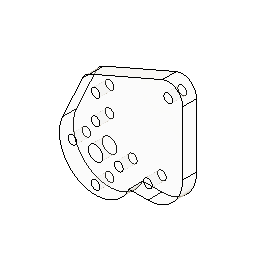
AssemblyHolderThrowerMotor v5 (Autodesk Fusion 360 archive; units mm, degrees)
design "ThrowerMotorJunction"
Autodesk Fusion 360 part; units mm, degrees
sketch "Sketch1" plane through (0, 0, 0) normal (0, 1, 0) x (1, 0, 0)
  circle A0 centre (0, 0) radius 8 construction
  circle A1 centre (0, 0) radius 9.5 construction
  circle A2 centre (0, 0) radius 14 construction
  circle A3 centre (0, 0) radius 18 construction
  line L0 (0, 0) -> (0, -18) construction
  line L1 (0, 0) -> (0, 52) construction
  line L2 (0, 0) -> (18, 0) construction
  line L3 (0, 0) -> (-18, 0) construction
  circle A4 centre (0, 0) radius 48 construction
  circle A5 centre (0, 0) radius 58 construction
  line L4 (0, 47) -> (-33.9853, 47) construction
  circle A6 centre (0, -9.5) radius 1.5
  circle A7 centre (-8, 0) radius 1.5
  circle A8 centre (8, 0) radius 1.5
  circle A9 centre (0, 9.5) radius 1.5
  circle A10 centre (18, 0) radius 1.5
  circle A11 centre (0, -18) radius 1.5
  line L5 (-50.3158, -28.85) -> (25, -28.85) construction
  circle A12 centre (25, -28.85) radius 1.5
  line L6 (-11.3632, -5.2083) -> (-4.1251, -21)
  line L7 (11.4564, 5) -> (18, 5)
  line L8 (30, -7) -> (30, -28.85)
  arc A13 (12.5, 0) -> (11.4564, 5) centre (0, 0) ccw construction
  arc A14 (11.4564, 5) -> (-11.3632, -5.2083) centre (0, 0) ccw
  arc A15 (0, -12.5) -> (12.5, 0) centre (0, 0) ccw construction
  arc A16 (-11.3632, -5.2083) -> (0, -12.5) centre (0, 0) ccw construction
  circle A17 centre (0, 0) radius 2.5
  arc A18 (30, -28.85) -> (23.0094, -33.4367) centre (25, -28.85) ccw construction
  arc A19 (23.0094, -33.4367) -> (30, -28.85) centre (25, -28.85) ccw
  line L9 (-1.9906, -22.5867) -> (23.0094, -33.4367)
  arc A20 (-1.9906, -22.5867) -> (-4.5453, -20.0833) centre (0, -18) ccw construction
  arc A21 (-4.5453, -20.0833) -> (-1.9906, -22.5867) centre (0, -18) ccw
  arc A22 (18, 5) -> (30, -7) centre (18, -7) ccw construction
  arc A23 (30, -7) -> (18, 5) centre (18, -7) ccw
  point P0 (0, 14)
  point P1 (0, 47)
  point P2 (-47.869, 32.75)
  point P3 (-42.1187, 39.875)
  point P4 (-50.8212, 27.95)
  point P5 (-55.4373, -17.05)
  point P6 (-53.7269, -21.85)
  point P7 (-50.3158, -28.85)
  point P8 (0, 9.5)
  point P9 (8, 0)
  point P10 (0, 12.5)
  dimension "d19" = 16
  dimension "d20" = 19
  dimension "d21" = 28
  dimension "d22" = 36
  dimension "d23" = 38
  dimension "d24" = 96
  dimension "d25" = 116
  dimension "d26" = 5
  dimension "d27" = 19.25
  dimension "d28" = 4.8
  dimension "d29" = 7.125
  dimension "d30" = 45
  dimension "d31" = 4.8
  dimension "d32" = 7
  dimension "d33" = 3
  dimension "d34" = 3
  dimension "d35" = 3
  dimension "d36" = 3
  dimension "d37" = 3
  dimension "d38" = 3
  dimension "d39" = 25
  dimension "d40" = 3
  dimension "d41" = 3
  dimension "d44" = 5
  dimension "d45" = 5
  dimension "d48" = 5
  dimension "d49" = 3
  dimension "d50" = 5
  dimension "d51" = 12
  constraint coincident A0.centre A1.centre
  constraint concentric A0 A2
  constraint concentric A1 A3
  constraint coincident A3 L0.end
  constraint vertical L0
  constraint parallel L0 L1
  constraint coincident A3 L2.end
  constraint horizontal L2
  constraint coincident A3 L3.end
  constraint parallel L2 L3
  constraint coincident A2 P0
  constraint coincident L1 P0
  constraint concentric A0 A4
  constraint concentric A3 A5
  constraint coincident L1 P1
  constraint coincident P1 L4.start
  constraint coincident A5 L4.end
  constraint perpendicular L1 L4
  constraint coincident A5 P2
  constraint coincident A5 P3
  constraint coincident A5 P4
  constraint coincident A5 P5
  constraint coincident A5 P6
  constraint coincident A5 P7
  constraint coincident A1 A6.centre
  constraint coincident L0 A6.centre
  constraint coincident A1 P8
  constraint coincident L1 P8
  constraint coincident A0 A7.centre
  constraint coincident L3 A7.centre
  constraint coincident A0 P9
  constraint coincident L2 P9
  constraint coincident P9 A8.centre
  constraint coincident P8 A9.centre
  constraint coincident L2.end A10.centre
  constraint coincident L0.end A11.centre
  constraint coincident P7 L5.start
  constraint horizontal L5
  constraint coincident L5.end A12.centre
  constraint concentric A3 A14
  constraint coincident L1 P10
  constraint coincident P10 A14
  constraint tangent L6 A14
  constraint horizontal L7
  constraint perpendicular L7 L8
  constraint coincident L2 A13.start
  constraint concentric A13 A14
  constraint coincident L0 A15.start
  constraint concentric A14 A15
  constraint concentric A14 A16
  constraint concentric A5 A17
  constraint concentric A12 A18
  constraint tangent L8 A18
  constraint concentric A18 A19
  constraint concentric A11 A20
  constraint tangent L6 A20
  constraint tangent A18 L9
  constraint tangent L9 A20
  constraint coincident L6 A20.end
  constraint concentric A20 A21
  constraint tangent L8 A22
  constraint tangent L7 A22
  constraint concentric A22 A23
  measures "d19" diameter of A0
  measures "d20" diameter of A1
  measures "d21" diameter of A2
  measures "d22" diameter of A3
  measures "d23" distance of L1.end P0
  measures "d24" diameter of A4
  measures "d25" diameter of A5
  measures "d26" distance of L1.end P1
  measures "d27" vertical distance of L1.end P2
  measures "d28" vertical distance of P2 P4
  measures "d29" vertical distance of P2 P3
  measures "d30" vertical distance of P4 P5
  measures "d31" vertical distance of P5 P6
  measures "d32" vertical distance of P6 P7
  measures "d33" diameter of A6
  measures "d34" diameter of A7
  measures "d35" diameter of A8
  measures "d36" diameter of A9
  measures "d37" diameter of A10
  measures "d38" diameter of A11
  measures "d39" horizontal distance of L0.end L5.end
  measures "d40" diameter of A12
  measures "d41" distance of P8 P10
  measures "d44" distance of L2.end L7
  measures "d45" distance of L5.end L8
  measures "d48" diameter of A17
  measures "d49" vertical distance of L6.end L0.end
  measures "d50" radius of A20
  measures "d51" distance of L8 A22.centre
extrude "Extrude1" add sketch "Sketch1" along normal blind 4.8

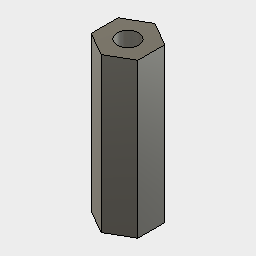
design "Spacer M3x18"
Autodesk Fusion 360 part; units mm, degrees
sketch "Sketch1" plane through (0, 0, 0) normal (0, 1, 0) x (1, 0, 0)
  line L0 (2.725, 1.5733) -> (0, 3.1466)
  line L1 (0, 3.1466) -> (-2.725, 1.5733)
  line L2 (-2.725, 1.5733) -> (-2.725, -1.5733)
  line L3 (-2.725, -1.5733) -> (0, -3.1466)
  line L4 (0, -3.1466) -> (2.725, -1.5733)
  line L5 (2.725, -1.5733) -> (2.725, 1.5733)
  circle A0 centre (0, 0) radius 1.25
  dimension "d1" = 2.5
  measures "d1" diameter of A0
extrude "Extrude1" add sketch "Sketch1" along normal blind 18

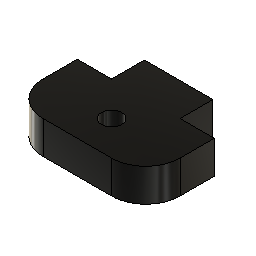
design "ThrowerLock"
Autodesk Fusion 360 part; units mm, degrees
sketch "Sketch1" plane through (0, 0, 0) normal (0, 0, 1) x (1, 0, 0)
  line L0 (-5, 9.8) -> (5, 9.8)
  line L1 (5, 9.8) -> (5, 5)
  line L2 (5, 5) -> (10, 5)
  line L3 (10, 5) -> (10, 0)
  line L4 (5, -5) -> (-5, -5)
  line L5 (-10, 0) -> (-10, 5)
  line L6 (-10, 5) -> (-5, 5)
  line L7 (-5, 5) -> (-5, 9.8)
  line L8 (0, 0) -> (0, 9.8) construction
  line L9 (0, 0) -> (10, 0) construction
  line L10 (0, 0) -> (0, -5) construction
  line L11 (-5, 5) -> (-5, 0) construction
  line L12 (0, 0) -> (-5, 0) construction
  circle A0 centre (0, 0) radius 1.5
  line L13 (-10, -5) -> (-10, 0) construction
  line L14 (-5, -5) -> (-10, -5) construction
  arc A1 (-5, -5) -> (-10, 0) centre (-5, 0) ccw construction
  arc A2 (-10, 0) -> (-5, -5) centre (-5, 0) ccw
  line L15 (10, -5) -> (5, -5) construction
  line L16 (10, 0) -> (10, -5) construction
  arc A3 (10, 0) -> (5, -5) centre (5, 0) ccw construction
  arc A4 (5, -5) -> (10, 0) centre (5, 0) ccw
  point P0 (0, 9.8)
  point P1 (0, -5)
  point P2 (5, 0)
  dimension "d1" = 10
  dimension "d2" = 5
  dimension "d3" = 4.8
  dimension "d5" = 3
  dimension "d6" = 10
  constraint horizontal L0
  constraint perpendicular L0 L1
  constraint perpendicular L1 L2
  constraint perpendicular L2 L3
  constraint perpendicular L1 L4
  constraint perpendicular L4 L5
  constraint perpendicular L5 L6
  constraint vertical L7
  constraint collinear L2 L6
  constraint midpoint L0 P0
  constraint coincident L8.start L9.start
  constraint coincident L0 P0
  constraint perpendicular L0 L8
  constraint coincident L3 L9.end
  constraint perpendicular L3 L9
  constraint coincident P0 L8.end
  constraint coincident L3.end L9.end
  constraint coincident L4 P1
  constraint perpendicular L4 L10
  constraint coincident P1 L10.end
  constraint perpendicular L6 L11
  constraint perpendicular L11 L12
  constraint coincident L11.end L12.end
  constraint tangent L4 A1
  constraint midpoint L9 P2
  constraint coincident P2 A3.centre
  constraint tangent L4 A3
  constraint perpendicular L4 L13
  constraint perpendicular L1 L14
  constraint tangent L14 A3
  constraint concentric A1 A2
  constraint perpendicular L1 L15
  constraint concentric A3 A4
  constraint parallel L3 L16
  constraint tangent L13 A2
  measures "d1" distance of L0.start L0.end
  measures "d2" distance of L1.end L2.end
  measures "d3" distance of L0.start L6.end
  measures "d5" diameter of A0
  measures "d6" distance of L4 L6
extrude "Extrude1" add sketch "Sketch1" along normal blind 4.8

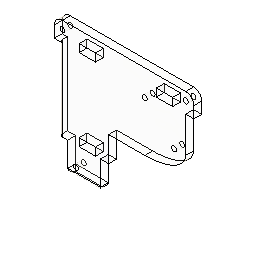
design "HolderThrowerMotor"
Autodesk Fusion 360 part; units mm, degrees
sketch "Sketch1" plane through (0, 0, 0) normal (0, 1, 0) x (1, 0, 0)
  circle A0 centre (0, 0) radius 14 construction
  circle A1 centre (0, 0) radius 48 construction
  circle A2 centre (0, 0) radius 58 construction
  circle A3 centre (0, 0) radius 68 construction
  line L0 (0, 0) -> (0, 52) construction
  line L1 (-9.7468, 47) -> (-49.1426, 47) construction
  line L2 (-35.0918, 32.75) -> (-59.5939, 32.75) construction
  line L3 (-39.023, 27.95) -> (-61.9903, 27.95) construction
  line L4 (-44.8698, -17.05) -> (-65.8278, -17.05) construction
  line L5 (-42.7385, -21.85) -> (-64.3939, -21.85) construction
  circle A4 centre (-50.3158, -28.85) radius 1.5
  circle A5 centre (-42.1187, 39.875) radius 1.5
  circle A6 centre (0, 0) radius 8 construction
  circle A7 centre (0, 0) radius 9.5 construction
  circle A8 centre (0, 0) radius 18 construction
  line L6 (0, 0) -> (18, 0) construction
  line L7 (0, 0) -> (0, -18) construction
  line L8 (0, 0) -> (-8, 0) construction
  circle A9 centre (0, -18) radius 1.5
  circle A10 centre (18, 0) radius 1.5
  circle A11 centre (0, -9.5) radius 1.5
  circle A12 centre (8, 0) radius 1.5
  circle A13 centre (0, 9.5) radius 1.5
  circle A14 centre (-8, 0) radius 1.5
  line L9 (-50.3158, -28.85) -> (25, -28.85) construction
  circle A15 centre (25, -28.85) radius 1.5
  line L10 (-50.3158, -33.85) -> (25, -33.85)
  line L11 (-55.3158, -21.85) -> (-55.3158, -28.85)
  arc A16 (-50.3158, -33.85) -> (-55.3158, -28.85) centre (-50.3158, -28.85) ccw construction
  arc A17 (-55.3158, -28.85) -> (-50.3158, -33.85) centre (-50.3158, -28.85) ccw
  line L12 (-52.1187, -21.85) -> (-52.1187, 27.95)
  line L13 (-52.1187, 27.95) -> (-47.1187, 27.95)
  line L14 (-52.1187, -21.85) -> (-55.3158, -21.85)
  line L15 (-47.1187, 27.95) -> (-47.1187, 44.875)
  line L16 (-47.1187, 44.875) -> (-27.1187, 44.875)
  line L17 (-27.1187, 44.875) -> (-27.1187, 27.95)
  line L18 (-27.1187, 27.95) -> (-22.1187, 27.95)
  line L19 (-40.1187, 27.95) -> (-30.1187, 27.95)
  line L20 (-30.1187, 27.95) -> (-30.1187, 23.15)
  line L21 (-30.1187, 23.15) -> (-40.1187, 23.15)
  line L22 (-40.1187, 23.15) -> (-40.1187, 27.95)
  line L23 (-30.1187, 27.95) -> (-27.1187, 27.95) construction
  line L24 (-40.1187, -21.85) -> (-30.1187, -21.85)
  line L25 (-30.1187, -21.85) -> (-30.1187, -26.65)
  line L26 (-30.1187, -26.65) -> (-40.1187, -26.65)
  line L27 (-40.1187, -26.65) -> (-40.1187, -21.85)
  line L28 (30, -28.85) -> (30, -21.85)
  line L29 (-30.1187, -21.85) -> (30, -21.85) construction
  arc A18 (30, -28.85) -> (25, -33.85) centre (25, -28.85) ccw construction
  arc A19 (25, -33.85) -> (30, -28.85) centre (25, -28.85) ccw
  line L30 (17, -21.85) -> (7, -21.85)
  line L31 (7, -21.85) -> (7, -26.65)
  line L32 (7, -26.65) -> (17, -26.65)
  line L33 (17, -26.65) -> (17, -21.85)
  line L34 (30, -21.85) -> (25, -21.85)
  line L35 (-22.1187, 27.95) -> (-22.1187, 12.5)
  line L36 (25, 0.0022) -> (25, -21.85)
  ellipse E0 centre (0, 0) end of major axis (25, 0) minor radius 12.5
  line L37 (-25, 0) -> (25, 0)
  line L38 (0, -12.5) -> (0, 12.5)
  line L39 (-22.1187, 12.5) -> (0, 12.5)
  line L40 (6.3048, 12.5) -> (25, 12.5) construction
  line L41 (0, 12.5) -> (6.3048, 12.5) construction
  line L42 (25, 12.5) -> (25, 0.0022) construction
  point P0 (0, 14)
  point P1 (-42.1187, 39.875)
  point P2 (-50.3158, -28.85)
  point P3 (0, -9.5)
  point P4 (8, 0)
  point P5 (0, 9.5)
  dimension "d1" = 28
  dimension "d2" = 96
  dimension "d3" = 116
  dimension "d4" = 136
  dimension "d5" = 38
  dimension "d6" = 5
  dimension "d7" = 19.25
  dimension "d8" = 4.8
  dimension "d9" = 45
  dimension "d10" = 4.8
  dimension "d11" = 7
  dimension "d12" = 7.125
  dimension "d13" = 3
  dimension "d14" = 3
  dimension "d15" = 16
  dimension "d16" = 19
  dimension "d17" = 36
  dimension "d18" = 3
  dimension "d19" = 3
  dimension "d20" = 3
  dimension "d21" = 3
  dimension "d22" = 3
  dimension "d23" = 3
  dimension "d24" = 25
  dimension "d25" = 3
  dimension "d26" = 10
  dimension "d27" = 10
  dimension "d28" = 10
  dimension "d29" = 5
  dimension "d30" = 5
  dimension "d31" = 5
  dimension "d32" = 10
  dimension "d33" = 4.8
  dimension "d34" = 8
  dimension "d35" = 10
  dimension "d36" = 4.8
  dimension "d37" = 12
  dimension "d38" = 7
  dimension "d39" = 10
  dimension "d40" = 4.8
  dimension "d42" = 5
  dimension "d43" = 3
  dimension "d44" = 12.5
  dimension "d45" = 25
  dimension "d51" = 8
  dimension "d53" = 12
  constraint coincident A0.centre A1.centre
  constraint concentric A0 A1
  constraint concentric A1 A2
  constraint concentric A0 A3
  constraint vertical L0
  constraint coincident L0 P0
  constraint coincident A0 P0
  constraint coincident A1 L1.start
  constraint coincident A3 L1.end
  constraint horizontal L1
  constraint coincident A1 L2.start
  constraint coincident A3 L2.end
  constraint parallel L1 L2
  constraint coincident A1 L3.start
  constraint coincident A3 L3.end
  constraint parallel L2 L3
  constraint coincident A1 L4.start
  constraint coincident A3 L4.end
  constraint parallel L3 L4
  constraint coincident A1 L5.start
  constraint coincident A3 L5.end
  constraint parallel L4 L5
  constraint coincident A2 P1
  constraint coincident A2 P2
  constraint coincident P2 A4.centre
  constraint coincident P1 A5.centre
  constraint concentric A1 A6
  constraint concentric A6 A8
  constraint coincident A8 L6.end
  constraint perpendicular L0 L6
  constraint coincident A8 L7.end
  constraint perpendicular L6 L7
  constraint coincident A6 L8.end
  constraint perpendicular L7 L8
  constraint coincident A7 P3
  constraint coincident L7 P3
  constraint coincident A6 P4
  constraint coincident L6 P4
  constraint coincident A7 P5
  constraint coincident L0 P5
  constraint coincident L7.end A9.centre
  constraint coincident L6.end A10.centre
  constraint coincident P3 A11.centre
  constraint coincident P4 A12.centre
  constraint coincident P5 A13.centre
  constraint coincident L8.end A14.centre
  constraint horizontal L9
  constraint coincident L9.end A15.centre
  constraint concentric A4 A16
  constraint concentric A15 A18
  constraint tangent L10 A18
  constraint parallel L9 L10
  constraint coincident L5 L11.start
  constraint tangent L11 A16
  constraint perpendicular L5 L11
  constraint concentric A16 A17
  constraint coincident L5 L12.start
  constraint coincident L3 L12.end
  constraint perpendicular L3 L12
  constraint perpendicular L12 L13
  constraint perpendicular L13 L15
  constraint perpendicular L15 L16
  constraint perpendicular L3 L17
  constraint perpendicular L17 L18
  constraint horizontal L19
  constraint vertical L20
  constraint horizontal L21
  constraint vertical L22
  constraint coincident L3 L19.start
  constraint perpendicular L17 L23
  constraint horizontal L24
  constraint vertical L25
  constraint horizontal L26
  constraint vertical L27
  constraint coincident L5 L24.start
  constraint perpendicular L9 L28
  constraint perpendicular L28 L29
  constraint concentric A18 A19
  constraint horizontal L30
  constraint vertical L31
  constraint horizontal L32
  constraint vertical L33
  constraint coincident L29 L30.start
  constraint perpendicular L28 L34
  constraint perpendicular L18 L35
  constraint perpendicular L35 L39
  constraint perpendicular L29 L36
  constraint concentric A0 E0
  constraint perpendicular L36 L37
  constraint coincident E0 L37.start
  constraint coincident E0 L37.end
  constraint coincident E0 L38.start
  constraint coincident E0 L38.end
  constraint coincident A0 L40.start
  constraint coincident E0 L36.start
  constraint perpendicular L29 L42
  constraint collinear L40 L41
  constraint collinear L39 L41
  measures "d1" diameter of A0
  measures "d2" diameter of A1
  measures "d3" diameter of A2
  measures "d4" diameter of A3
  measures "d5" distance of L0.end P0
  measures "d6" distance of L0.end L1
  measures "d7" distance of L0.end L2
  measures "d8" distance of L2 L3
  measures "d9" distance of L3 L4
  measures "d10" distance of L4 L5
  measures "d11" distance of L5 P2
  measures "d12" distance of L2 P1
  measures "d13" diameter of A4
  measures "d14" diameter of A5
  measures "d15" diameter of A6
  measures "d16" diameter of A7
  measures "d17" diameter of A8
  measures "d18" diameter of A9
  measures "d19" diameter of A10
  measures "d20" diameter of A11
  measures "d21" diameter of A12
  measures "d22" diameter of A13
  measures "d23" diameter of A14
  measures "d24" horizontal distance of A0.centre L9.end
  measures "d25" diameter of A15
  measures "d26" diameter of A16
  measures "d27" diameter of A18
  measures "d28" distance of P1 L12
  measures "d29" distance of L12.end L13.end
  measures "d30" distance of L17.end L18.end
  measures "d31" distance of P1 L16
  measures "d32" distance of L19.start L19.end
  measures "d33" distance of L19.start L21.end
  measures "d34" distance of L18.end L20
  measures "d35" distance of L24.start L24.end
  measures "d36" distance of L24.start L26.end
  measures "d37" distance of L12 L27
  measures "d38" distance of L28.start L28.end
  measures "d39" distance of L30.start L30.end
  measures "d40" distance of L30.start L32.end
  measures "d42" distance of L28.end L34.end
  measures "d43" distance of P5 L39
  measures "d45" distance of E0
  measures "d51" distance of L9.end L33
  measures "d53" distance of L12 L22
extrude "Extrude1" add sketch "Sketch1" along normal blind 4.8 contours A10 A11 A12 E0 L37 L38 | A10 A12 A13 L36 E0 L37 L38 | L10 L11 A17 L12 L13 L14 L15 L16 L17 L18 L28 A19 L34 L35 L36 E0 L39 | A12 L37 | A12 L37 | A11 A14 E0 L37 L38 | A13 A14 E0 L37 L38 | A11 L38 | A11 L38 | A13 L38 | A13 L38 | A14 L37 | A14 L37
fillet "Fillet1" radius 2 4 edges at (-47.1187, 2.4, -44.875) (-37.1187, 4.8, -44.875) (-37.1187, 0, -44.875) (-27.1187, 2.4, -44.875)
fillet "Fillet2" radius 2 1 edges at (-52.1187, 0, -3.05)
